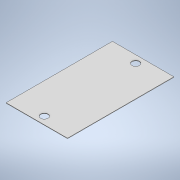
# Autodesk Inventor part: base ultrasonido
Saved by Autodesk Inventor 2021 (Build 250183000, 183)
## iProperties
Created: 2024-01-19
Part Number: base ultrasonido
Material: Generic
Document SubType Name: Modeling
Designer: MARCO BRAVO
Density: 1 g/cm^3
Appearance: Default
Author: MARCO BRAVO
Autodesk Inventor part; units mm, degrees
ref_plane "YZ Plane" through (0, 0, 0) normal (1, 0, 0) x (0, 1, 0)
ref_plane "XZ Plane" through (0, 0, 0) normal (0, 1, 0) x (-1, 0, 0)
ref_plane "XY Plane" through (0, 0, 0) normal (0, 0, 1) x (1, 0, 0)
sketch "Sketch1" plane through (0, 0, 0) normal (0, 1, 0) x (-1, 0, 0)
  line L0 (-266.0977, 629.1478) -> (143.9023, 629.1478)
  line L1 (143.9023, 629.1478) -> (143.9023, -80.8522)
  line L2 (143.9023, -80.8522) -> (-266.0977, -80.8522)
  line L3 (-266.0977, -80.8522) -> (-266.0977, 629.1478)
  circle A0 centre (-61.0977, 579.1478) radius 25
  circle A1 centre (-61.0977, -30.8522) radius 25
  point P0 (0, 0)
  dimension "d0" = 710
  dimension "d1" = 410
  dimension "d4" = 50
  dimension "d5" = 50
  constraints: 8 end point, 2 centre point, 2 parallel, 1 horizontal, 1 perpendicular
  measures "d0" distance of L0.end L1.end
  measures "d1" distance of L1.end L2.end
  measures "d4" diameter of A0
  measures "d5" diameter of A1
extrude "Extrusion1" add sketch "Sketch1" along normal blind 3
body "Solid1"
